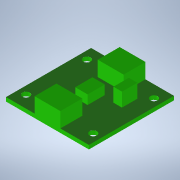
# Autodesk Inventor part: Prozessorboard
Saved by Autodesk Inventor 2020.2 (Build 242310000, 310)
## iProperties
Created: 2020-02-12
Part Number: Prozessorboard
Material: Generisch
Document SubType Name: Modeling
Designer: Max
Density: 1 g/cm^3
Appearance: Vorgabe
Author: Max
Autodesk Inventor part; units mm, degrees
ref_plane "YZ Plane" through (0, 0, 0) normal (1, 0, 0) x (0, 1, 0)
ref_plane "XZ Plane" through (0, 0, 0) normal (0, 1, 0) x (-1, 0, 0)
ref_plane "XY Plane" through (0, 0, 0) normal (0, 0, 1) x (1, 0, 0)
sketch "Skizze1" plane through (0, 0, 0) normal (0, 1, 0) x (-1, 0, 0)
  line L0 (17.05, 17.5) -> (-17.05, 17.5)
  line L1 (-17.05, 17.5) -> (-17.05, -17.5)
  line L2 (-17.05, -17.5) -> (17.05, -17.5)
  line L3 (17.05, -17.5) -> (17.05, 17.5)
  point P0 (0, 0)
  dimension "d0" = 35
  dimension "d1" = 34.1
  dimension "d2" = 17.5
  dimension "d3" = 17.05
  constraints: 8 end point, 2 parallel, 1 horizontal, 1 perpendicular
  measures "d0" distance of L2.end L0.start
  measures "d1" distance of L0.start L0.end
  measures "d2" distance from line of point (0, 0) L0
  measures "d3" distance from line of point (0, 0) L3
extrude "Extrusion1" add sketch "Skizze1" along normal blind 1.6
sketch "Skizze3" plane through (0, 1.6, 0) normal (0, 1, 0) x (1, 0, 0)
  line L0 (-17.05, 17.5) -> (-17.05, -17.5) projected
  line L1 (17.05, -17.5) -> (17.05, 17.5) projected
  line L2 (-21.1922, 0) -> (21.294, 0)
  point P0 (0, 0)
  point P1 (-13.8, -12.5)
  point P2 (13.8, 12.5)
  point P3 (13.8, -12.5)
  point P4 (-13.8, 12.5)
  dimension "d13" = 3.25
  dimension "d15" = 3.25
  dimension "d16" = 25
  dimension "d18" = 25
  constraints: 2 end point, 2 symmetric about line, 1 horizontal, 1 point on line
  measures "d13" distance from line of L0 point (-13.8, -12.5)
  measures "d15" distance from line of L1 point (13.8, 12.5)
  measures "d16" distance of point (13.8, 12.5) point (13.8, -12.5)
  measures "d18" distance of point (-13.8, 12.5) point (-13.8, -12.5)
hole "Bohrung2" at (-13.8, 1.6, 12.5) at (13.8, 1.6, -12.5) at (13.8, 1.6, 12.5) at (-13.8, 1.6, -12.5) direction (0, -1, 0) diameter 3 end through all
sketch "Skizze4" plane through (0, 1.6, 0) normal (0, 1, 0) x (1, 0, 0)
  line L0 (17.05, 17.5) -> (-17.05, 17.5) projected
  line L1 (-5.3, 17.5) -> (5.3, 17.5)
  line L2 (5.3, 17.5) -> (5.3, 8.5)
  line L3 (5.3, 8.5) -> (-5.3, 8.5)
  line L4 (-5.3, 8.5) -> (-5.3, 17.5)
  line L5 (0, -9.1387) -> (0, 30.8608)
  line L6 (-26.2563, 0) -> (26.186, 0)
  line L7 (-17.05, -17.5) -> (17.05, -17.5) projected
  line L8 (-5.3, -17.5) -> (5.3, -17.5)
  line L9 (5.3, -17.5) -> (5.3, -8.5)
  line L10 (5.3, -8.5) -> (-5.3, -8.5)
  line L11 (-5.3, -8.5) -> (-5.3, -17.5)
  point P0 (0, 0)
  dimension "d26" = 9
  dimension "d27" = 10.6
  constraints: 20 end point, 4 parallel, 3 horizontal, 3 point on line, 2 equal length, 2 perpendicular, 1 vertical, 2 other
  measures "d26" distance between parallel lines of L0 L3
  measures "d27" distance between parallel lines of L2 L4
extrude "Extrusion2" add sketch "Skizze4" along normal blind 6.2
sketch "Skizze5" plane through (0, 1.6, 0) normal (0, 1, 0) x (1, 0, 0)
  line L0 (10.55, 2.6) -> (7.05, 2.6)
  line L1 (7.05, 2.6) -> (7.05, 8.9)
  line L2 (7.05, 8.9) -> (10.55, 8.9)
  line L3 (10.55, 8.9) -> (10.55, 2.6)
  line L4 (17.05, -17.5) -> (17.05, 17.5) projected
  line L5 (17.05, 17.5) -> (5.3, 17.5) projected
  point P0 (0, 0)
  dimension "d32" = 6.3
  dimension "d33" = 3.5
  dimension "d34" = 6.5
  dimension "d35" = 8.6
  constraints: 8 end point, 2 parallel, 1 horizontal, 1 perpendicular
  measures "d32" distance between parallel lines of L2 L0
  measures "d33" distance of L1.end L2.end
  measures "d34" distance between parallel lines of L4 L3
  measures "d35" distance between parallel lines of L5 L2
extrude "Extrusion3" add sketch "Skizze5" along normal blind 5.7
sketch "Skizze6" plane through (0, 1.6, 0) normal (0, 1, 0) x (1, 0, 0)
  line L0 (-2.55, -3.55) -> (2.55, -3.55)
  line L1 (2.55, -3.55) -> (2.55, 3.55)
  line L2 (2.55, 3.55) -> (-2.55, 3.55)
  line L3 (-2.55, 3.55) -> (-2.55, -3.55)
  line L4 (-17.05, 17.5) -> (-17.05, -17.5) projected
  line L5 (5.3, 17.5) -> (-5.3, 17.5) projected
  point P0 (0, 0)
  dimension "d38" = 7.1
  dimension "d39" = 5.1
  dimension "d40" = 14.5
  dimension "d41" = 13.95
  constraints: 8 end point, 2 parallel, 1 horizontal, 1 perpendicular
  measures "d38" distance of L2.end L0.start
  measures "d39" distance of L1.end L2.end
  measures "d40" distance between parallel lines of L4 L3
  measures "d41" distance between parallel lines of L5 L2
extrude "Extrusion4" add sketch "Skizze6" along normal blind 3.8
